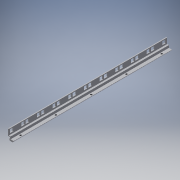
# Autodesk Inventor part: TBD
Saved by Autodesk Inventor 2018 (Build 220105000, 105)
## iProperties
Created: 2004-11-19
Material: Aluminum-6061
Document SubType Name: Modeling
Designer: Autodesk, Inc.
Manufacturer: Standard
Standards Organization: Custom
Stock Number: 12-109M
Catalog Web Link: http://www.parker.com/ead/cm1.asp?cmid=809
Description: 19" RACK ANGLE
Vendor: PARKER IPS
Part Number: TBD
Mass: 126.265 g
Surface Area: 389.073 cm^2
Volume: 46.5923 cm^3
Density: 2.71 g/cm^3
Appearance: Aluminum - Flat
CAGE: 1LJX3
Dept. ID: Product Design
Description #2: ---
Finish #1: ---
Finish #2: ---
Material ID: ---
Project Number: ---
Author: Autodesk, Inc.
Autodesk Inventor part; units mm, degrees
ref_plane "YZ Plane" through (0, 0, 0) normal (1, 0, 0) x (0, 1, 0)
ref_plane "XZ Plane" through (0, 0, 0) normal (0, 1, 0) x (-1, 0, 0)
ref_plane "XY Plane" through (0, 0, 0) normal (0, 0, 1) x (1, 0, 0)
sketch "Sketch1" plane through (0, 0, 0) normal (0, 0, 1) x (1, 0, 0)
  line L0 (-2.8679, 4.0958) -> (0, 0)
  line L1 (0, 0) -> (7.7642, 0)
  line L2 (7.7642, 0) -> (10.6321, 4.0958)
  line L3 (10.6321, 4.0958) -> (10.6321, 4.7)
  line L4 (10.6321, 4.7) -> (1.7321, 4.7)
  line L5 (1.7321, 4.7) -> (1.7321, 11.5)
  line L6 (1.7321, 11.5) -> (-3.2679, 11.5)
  line L7 (-3.2679, 11.5) -> (-3.2679, 27.5)
  line L8 (-3.2679, 27.5) -> (-5.7679, 27.5)
  line L9 (-5.7679, 27.5) -> (-5.7679, 9.5)
  line L10 (-5.7679, 9.5) -> (0.0321, 9.5)
  line L11 (0.0321, 9.5) -> (0.0321, 4.7)
  line L12 (0.0321, 4.7) -> (-2.8679, 4.7)
  line L13 (-2.8679, 4.7) -> (-2.8679, 4.0958)
  constraints: 28 end point, 6 horizontal, 6 vertical, 16 other
extrude "Extrusion1" add sketch "Sketch1" against normal blind 448.75
sketch "Sketch2" plane through (1.7321, 4.7, 0) normal (0, 1, 0) x (1, 0, 0)
  line L0 (8.9, 0) -> (0, 0) projected
  point P0 (4.45, 24)
  point P1 (4.45, 0)
  dimension "d2" = 24
  constraints: 1 midpoint, 1 vertical alignment
  measures "d2" distance from line of L0 point (4.45, 24)
hole "Hole1" at (6.1821, 4.7, -24) direction (0, -1, 0) diameter 4.917 end through all thread size "M6x1" class "6H" standard "ANSI Metric M Profile"
pattern_linear "Rectangular Pattern1" count 5 spacing 100 along (0, 0, -1) of "Hole1"
sketch "Sketch3" plane through (-3.2679, 11.5, 0) normal (1, 0, 0) x (0, 0, -1)
  line L0 (3.25, 13.75) -> (12.75, 13.75)
  line L1 (12.75, 13.75) -> (12.75, 4.25)
  line L2 (12.75, 4.25) -> (3.25, 4.25)
  line L3 (3.25, 4.25) -> (3.25, 13.75)
  line L4 (8, 13.75) -> (8, 4.25) construction
  line L5 (0, 0) -> (0, 16) construction
  line L6 (3.25, 9) -> (12.75, 9) construction
  line L7 (0, -2) -> (448.75, -2) construction
  dimension "d13" = 9.5
  dimension "d14" = 8
  dimension "d15" = 11
  constraints: 12 end point, 4 midpoint, 2 parallel, 2 perpendicular, 1 horizontal
  measures "d13" distance of L0.end L1.end
  measures "d14" distance between parallel lines of L4 L5
  measures "d15" distance between parallel lines of L7 L6
extrude "12-109M" cut sketch "Sketch3" against normal through all
pattern_linear "Rectangular Pattern2" count 2 spacing 31.75 along (0, 0, -1) count 10 spacing 44.45 along (0, 0, -1) of "12-109M"
body "Solid1"
